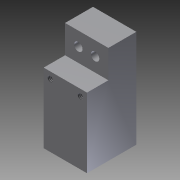
# Autodesk Inventor part: X+Z axis home sensor block
Saved by Autodesk Inventor 2011 (Build 150239000, 239)
## iProperties
Created: 2014-04-04
Part Number: X+Z axis home sensor block
Document SubType Name: Modeling
Designer: Devon
Density: 1 g/cm^3
Author: Devon
Autodesk Inventor part; units mm, degrees
ref_plane "YZ Plane" through (0, 0, 0) normal (1, 0, 0) x (0, 1, 0)
ref_plane "XZ Plane" through (0, 0, 0) normal (0, 1, 0) x (-1, 0, 0)
ref_plane "XY Plane" through (0, 0, 0) normal (0, 0, 1) x (1, 0, 0)
sketch "Sketch1" plane through (0, 0, 0) normal (0, 0, 1) x (1, 0, 0)
  line L0 (-24.6491, 25.3024) -> (-4.9641, 25.3024)
  line L1 (-4.9641, 25.3024) -> (-4.9641, -19.1476)
  line L2 (-4.9641, -19.1476) -> (-24.6491, -19.1476)
  line L3 (-24.6491, -19.1476) -> (-24.6491, 25.3024)
  point P0 (0, 0)
  dimension "d0" = 19.685
  dimension "d1" = 44.45
  constraints: 8 end point, 2 parallel, 1 horizontal, 1 perpendicular
  measures "d0" distance of L1.end L2.end
  measures "d1" distance of L0.end L1.end
extrude "Extrusion1" add sketch "Sketch1" along normal blind 12.7
sketch "Sketch2" plane through (0, 0, 12.7) normal (0, 0, 1) x (1, 0, 0)
  line L0 (-4.9641, 25.3024) -> (-4.9641, -19.1476) projected
  line L1 (-24.6491, -19.1476) -> (-4.9641, -19.1476)
  line L2 (-4.9641, -19.1476) -> (-4.9641, 12.577)
  line L3 (-4.9641, 12.577) -> (-24.6491, 12.577)
  line L4 (-24.6491, 12.577) -> (-24.6491, -19.1476)
  point P0 (0, 0)
  dimension "d4" = 31.7246
  constraints: 8 end point, 2 parallel, 1 horizontal, 1 perpendicular, 1 point on line
  measures "d4" distance of L2.end L1.end
extrude "Extrusion2" add sketch "Sketch2" along normal blind 9.7282
sketch "Sketch3" plane through (0, 0, 22.4282) normal (0, 0, 1) x (1, 0, 0)
  line L0 (-24.6491, 12.577) -> (-4.9641, 12.577) projected
  line L1 (-4.9641, 12.577) -> (-7.9613, 12.577)
  line L2 (-7.9613, 12.577) -> (-7.9613, 9.5798)
  line L3 (-24.6491, 12.577) -> (-21.6519, 12.577)
  line L4 (-21.6519, 12.577) -> (-21.6519, 9.5798)
  point P0 (0, 0)
  dimension "d7" = 2.9972
  dimension "d8" = 2.9972
  dimension "d9" = 2.9972
  dimension "d10" = 2.9972
  constraints: 8 end point, 2 perpendicular, 2 point on line
  measures "d7" distance of L0.end L1.end
  measures "d8" distance of L1.end L2.end
  measures "d9" distance of L0.start L3.end
  measures "d10" distance of L3.end L4.end
hole "Hole1" at (-21.6519, 9.5798, 22.4282) at (-7.9613, 9.5798, 22.4282) direction (0, 0, -1) diameter 2.4892 depth 12.7 tip angle 118
sketch "Sketch4" plane through (0, 0, 12.7) normal (0, 0, 1) x (1, 0, 0)
  line L0 (-24.6491, 12.577) -> (-4.9641, 12.577) projected
  line L1 (-24.6491, 25.3024) -> (-4.9641, 25.3024) projected
  line L2 (-14.8066, 25.3024) -> (-14.8066, 12.577)
  line L3 (-14.8066, 18.9397) -> (-10.9966, 18.9397)
  line L4 (-14.8066, 18.9397) -> (-18.6166, 18.9397)
  point P0 (0, 0)
  dimension "d18" = 3.81
  dimension "d19" = 3.81
  constraints: 6 end point, 3 midpoint, 1 collinear, 1 perpendicular
  measures "d18" distance of L3.start L3.end
  measures "d19" distance of L3.start L4.end
hole "Hole2" at (-10.9966, 18.9397, 12.7) at (-18.6166, 18.9397, 12.7) direction (0, 0, -1) diameter 3.81 depth 12.7 tip angle 118 clearance for "Flat Head Machine Screw (82)" size "#6" standard "Ansi Unified Screw Threads"
body "Solid1"
